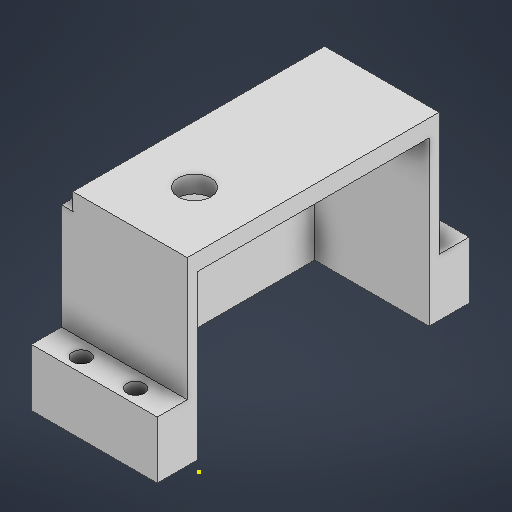
# Autodesk Inventor part: servo_horni_kloub
Saved by Autodesk Inventor 2026 (Build 300175000, 175)
## iProperties
Created: 2025-04-11
Part Number: servo_horni_kloub
Material: Generic
Document SubType Name: Modeling
Designer: janpa
Density: 1 g/cm^3
Appearance: Default
Author: janpa
Autodesk Inventor part; units mm, degrees
ref_plane "YZ Plane" through (0, 0, 0) normal (1, 0, 0) x (0, 1, 0)
ref_plane "XZ Plane" through (0, 0, 0) normal (0, 1, 0) x (-1, 0, 0)
ref_plane "XY Plane" through (0, 0, 0) normal (0, 0, 1) x (1, 0, 0)
sketch "Sketch1" plane through (0, 0, 0) normal (0, 1, 0) x (-1, 0, 0)
  line L0 (0, 0) -> (24, 0)
  line L1 (24, 0) -> (24, -44)
  line L2 (24, -44) -> (0, -44)
  line L3 (0, -44) -> (0, 0)
  line L4 (2, -1.75) -> (22, -1.75)
  line L5 (22, -1.75) -> (22, -42.25)
  line L6 (22, -42.25) -> (2, -42.25)
  line L7 (2, -42.25) -> (2, -1.75)
  line L8 (22, -42.25) -> (22, -44)
  line L9 (22, -1.75) -> (22, 0)
  line L10 (2, 0) -> (2, -44)
  dimension "d0" = 24
  dimension "d1" = 44
  dimension "d2" = 20
  dimension "d3" = 40.5
  dimension "d4" = 2
  dimension "d5" = 1.75
  constraints: 22 end point, 5 point on line, 4 parallel, 4 perpendicular, 2 horizontal
  measures "d0" distance of L1.end L2.end
  measures "d1" distance of L0.end L1.end
  measures "d2" distance of L5.end L6.end
  measures "d3" distance of L4.end L5.end
  measures "d4" distance between parallel lines of L1 L5
  measures "d5" distance between parallel lines of L2 L6
extrude "Extrusion1" add sketch "Sketch1" along normal blind 3 contours L0 L9 L4 L10 | L4 L5 L6 L7 | L10 L6 L8 L2
extrude "Extrusion2" add sketch "Sketch1" against normal blind 28.5 contours L0 L9 L4 L10 | L0 L1 L2 L8 L5 L9 | L10 L6 L8 L2
sketch "Sketch2" plane through (0, -28.5, 0) normal (0, -1, 0) x (1, 0, 0)
  point P0 (0, 0)
sketch "Sketch3" plane through (0, 0, 0) normal (0, -1, 0) x (1, 0, 0)
  circle A0 centre (-12, -11.25) radius 2.85
  line L0 (-22, -1.75) -> (-2, -1.75) projected
  line L1 (-2, -1.75) -> (-2, -42.25) projected
  point P0 (0, 0)
  dimension "d10" = 5.7
  dimension "d11" = 9.5
  dimension "d12" = 10
  constraints: 1 centre point
  measures "d10" diameter of A0
  measures "d11" distance from line of L0 A0.centre
  measures "d12" distance from line of A0.centre L1
extrude "Extrusion3" cut sketch "Sketch3" against normal blind 28.5
sketch "Sketch5" plane through (0, -28.5, 0) normal (0, -1, 0) x (1, 0, 0)
  line L0 (0, -44) -> (0, 0) projected
  line L1 (0, -42.25) -> (-24, -42.25)
  line L2 (-24, -42.25) -> (-24, -49.25)
  line L3 (-24, -49.25) -> (0, -49.25)
  line L4 (-2, -42.25) -> (-22, -42.25) projected
  line L5 (0, -22) -> (2.0773, -22)
  line L6 (0, -1.75) -> (-24, -1.75)
  line L7 (-24, -1.75) -> (-24, 5.25)
  line L8 (-24, 5.25) -> (-2, 5.25)
  line L9 (-2, -1.75) -> (-22, -1.75)
  circle A0 centre (-17.75, -46.8) radius 1.5
  circle A1 centre (-8.25, -46.8) radius 1.5
  circle A2 centre (-17.75, 2.8) radius 1.5
  circle A3 centre (-8.25, 2.8) radius 1.5
  line L10 (-24, 0) -> (-24, -44) projected
  line L11 (-2, 5.25) -> (-2, -49.25)
  point P0 (-2, -1.75)
  dimension "d15" = 7
  dimension "d16" = 3
  dimension "d19" = 9.5
  dimension "d22" = 49.6
  dimension "d25" = 2.45
  dimension "d26" = 6.25
  dimension "d27" = 2.45
  constraints: 14 end point, 5 symmetric about line, 4 centre point, 4 horizontal, 2 equal radius, 2 point on line, 2 vertical alignment, 1 collinear, 1 midpoint, 1 parallel, 1 perpendicular, 1 vertical, 8 other
  measures "d15" distance of L3.start L1.end
  measures "d16" diameter of A0
  measures "d19" distance of A0.centre A1.centre
  measures "d22" distance of A0.centre A2.centre
  measures "d25" distance from line of L3 A0.centre
  measures "d27" distance from line of L8 A2.centre
extrude "Extrusion4" add sketch "Sketch5" against normal blind 10 contours L11 L3 L2 L1 | L6 L7 L8 L11
body "Solid1"
